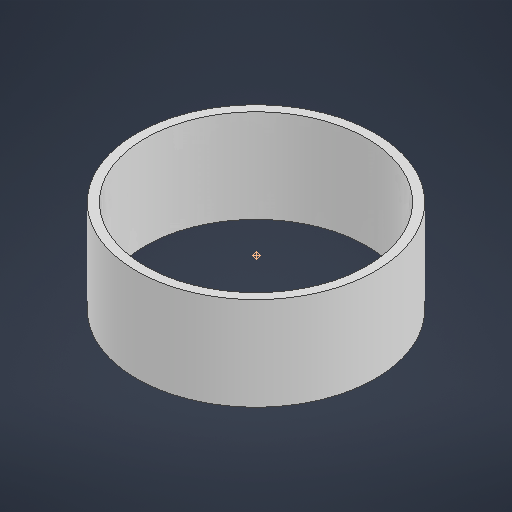
# Autodesk Inventor part: Outboard_Bearing_Housing
Saved by Autodesk Inventor 2026.1 (Build 301233000, 233)
## iProperties
Created: 2026-09-19
Part Number: Outboard_Bearing_Housing
Material: Generic
Document SubType Name: Modeling
Designer: share
Density: 1 g/cm^3
Appearance: Default
Author: share
Autodesk Inventor part; units mm, degrees
sketch "Sketch2" plane through (0, 0, 0) normal (0, 1, 0) x (-1, 0, 0)
  circle A0 centre (0, 0) radius 15.0812
  circle A1 centre (0, 0) radius 16.25
  dimension "d7" = 30.1625
  dimension "d16" = 32.5
  dimension "d17" = 1.1687
  constraints: 2 centre point, 2 coincident
  measures "d7" diameter of A0
  measures "d16" diameter of A1
  measures "d17" radial gap between concentric circles of A1 A0
extrude "Extrusion2" add sketch "Sketch2" along normal mid plane 12.7
equation "\"Bearing_OD\" = 30.1625"
body "Solid2"
